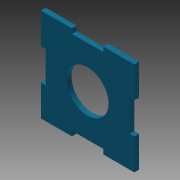
# Autodesk Inventor part: Side A
Saved by Autodesk Inventor 2014 (Build 180170000, 170)
## iProperties
Created: 2014-11-21
Part Number: Side A
Material: Generic
Document SubType Name: Modeling
Designer: JLM
Density: 1 g/cm^3
Appearance: Default
Author: JLM
Autodesk Inventor part; units mm, degrees
ref_plane "YZ Plane" through (0, 0, 0) normal (1, 0, 0) x (0, 1, 0)
ref_plane "XZ Plane" through (0, 0, 0) normal (0, 1, 0) x (-1, 0, 0)
ref_plane "XY Plane" through (0, 0, 0) normal (0, 0, 1) x (1, 0, 0)
sketch "Sketch1" plane through (0, 0, 0) normal (0, 0, 1) x (1, 0, 0)
  line L0 (-28.321, -28.321) -> (28.321, -28.321)
  line L1 (28.321, -28.321) -> (28.321, 28.321)
  line L2 (28.321, 28.321) -> (-28.321, 28.321)
  line L3 (-28.321, 28.321) -> (-28.321, -28.321)
  line L4 (-28.321, -28.321) -> (28.321, 28.321) construction
  line L5 (28.321, -28.321) -> (-28.321, 28.321) construction
  point P0 (0, 0)
  dimension "d0" = 56.642
  dimension "d1" = 56.642
  constraints: 12 end point, 2 midpoint, 2 parallel, 1 horizontal, 1 perpendicular
  measures "d0" distance of L2.end L1.end
  measures "d1" distance of L1.end L0.end
extrude "Extrusion1" add sketch "Sketch1" against normal blind 2.921
sketch "Sketch2" plane through (0, 0, 0) normal (0, 0, 1) x (1, 0, 0)
  line L0 (-10.2341, 28.321) -> (-9.525, 28.321)
  line L1 (-9.525, 28.321) -> (-9.525, 25.4)
  line L2 (-9.525, 25.4) -> (9.525, 25.4)
  line L3 (9.525, 25.4) -> (9.525, 28.321)
  line L4 (-9.525, 28.321) -> (9.525, 28.321)
  line L5 (-9.525, -28.321) -> (9.525, -28.321)
  line L6 (9.525, -28.321) -> (9.525, -25.4)
  line L7 (9.525, -25.4) -> (-9.525, -25.4)
  line L8 (-9.525, -25.4) -> (-9.525, -28.321)
  line L9 (-28.321, 9.525) -> (-25.4, 9.525)
  line L10 (-25.4, 9.525) -> (-25.4, -9.525)
  line L11 (-25.4, -9.525) -> (-28.321, -9.525)
  line L12 (-28.321, -9.525) -> (-28.321, 9.525)
  line L13 (28.321, 9.525) -> (25.4, 9.525)
  line L14 (25.4, 9.525) -> (25.4, -9.525)
  line L15 (25.4, -9.525) -> (28.321, -9.525)
  line L16 (28.321, -9.525) -> (28.321, 9.525)
  line L17 (28.321, -28.321) -> (28.321, 28.321) projected
  line L18 (-28.321, 28.321) -> (-28.321, -28.321) projected
  line L19 (-28.321, -28.321) -> (28.321, -28.321) projected
  line L20 (28.321, 28.321) -> (-28.321, 28.321) projected
  line L21 (-28.321, 28.321) -> (-28.321, -28.321) projected
  dimension "d4" = 2.921
  dimension "d5" = 19.05
  dimension "d17" = 19.05
  dimension "d18" = 2.921
  dimension "d19" = 2.921
  dimension "d20" = 19.05
  dimension "d34" = 2.921
  dimension "d35" = 19.05
  dimension "d47" = 18.796
  dimension "d48" = 18.796
  dimension "d49" = 18.796
  dimension "d50" = 18.796
  dimension "d51" = 18.796
  dimension "d52" = 18.796
  dimension "d54" = 18.796
  dimension "d55" = 18.796
  constraints: 34 end point, 6 parallel, 5 perpendicular, 4 collinear, 3 horizontal
  measures "d4" distance of L0.end L1.end
  measures "d5" distance of L1.end L2.end
  measures "d17" distance of L7.end L6.end
  measures "d18" distance of L6.end L5.end
  measures "d19" distance of L10.end L11.end
  measures "d20" distance of L9.end L10.end
  measures "d34" distance of L15.end L14.end
  measures "d35" distance of L14.end L13.end
  measures "d47" distance between parallel lines of L18 L1
  measures "d48" distance between parallel lines of L17 L3
  measures "d49" distance between parallel lines of L20 L9
  measures "d50" distance between parallel lines of L21 L8
  measures "d51" distance between parallel lines of L19 L15
  measures "d52" distance between parallel lines of L19 L11
  measures "d54" distance between parallel lines of L20 L13
  measures "d55" distance between parallel lines of L17 L6
extrude "Extrusion3" cut sketch "Sketch2" against normal blind 25.4 contours L4 L3 L2 L1 | L9 L10 L11 L12 | L16 L15 L14 L13 | L8 L7 L6 L5
hole "Hole1" at (0, 0, 0) direction (0, 0, -1) diameter 25.4 end through all
equation "\"d1\" = d0"
equation "\"d17\" = d5"
equation "\"d18\" = d4"
equation "\"d19\" = d4"
equation "\"d20\" = d5"
equation "\"d34\" = d4"
equation "\"d35\" = d5"
equation "\"d47\" = -0.5 * d5 + 0.5 * d0"
equation "\"d49\" = d47"
equation "\"d50\" = d47"
equation "\"d51\" = d47"
equation "\"d23\" = 0.5 * d0"
equation "\"d53\" = 0.5 * d0"
body "Solid1"
